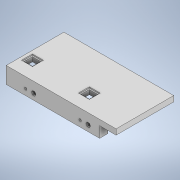
# Autodesk Inventor part: side_bumper_lower_R_new
Saved by Autodesk Inventor 2020 (Build 240168000, 168)
## iProperties
Created: 2022-10-31
Part Number: side_bumper_lower_R_new
Material: 일반
Document SubType Name: Modeling
Designer: SeungJin
Density: 1 g/cm^3
Appearance: 기본값
Author: SeungJin
Autodesk Inventor part; units mm, degrees
ref_plane "YZ Plane" through (0, 0, 0) normal (1, 0, 0) x (0, 1, 0)
ref_plane "XZ Plane" through (0, 0, 0) normal (0, 1, 0) x (-1, 0, 0)
ref_plane "작업 평면1" through (18.73, 22.5444, -43) normal (0, 0, -1) x (-1, 0, 0)
sketch "스케치1" plane through (18.73, 22.5444, -43) normal (0, 0, -1) x (-1, 0, 0)
  circle A0 centre (15, -32.544) radius 4
  circle A1 centre (215, -32.544) radius 4
  circle A2 centre (164.635, -19) radius 2.25
  circle A3 centre (65.365, -19) radius 2.25
  line L0 (230, 0) -> (230, -40)
  line L1 (0, 0) -> (230, 0)
  line L2 (0, -40) -> (0, 0)
  line L3 (230, -40) -> (0, -40)
  line L4 (230, -40) -> (0, -40)
  line L5 (0, 0) -> (230, 0)
  line L6 (200, -40) -> (200, 0)
  line L7 (30, -40) -> (30, 0)
  line L8 (230, -10) -> (0, -10)
  point P0 (200, 0)
  point P1 (30, -10)
  dimension "d5" = 40
  dimension "d6" = 230
  dimension "d7" = 15
  dimension "d8" = 7.456
  dimension "d9" = 7.456
  dimension "d10" = 15
  dimension "d11" = 19
  dimension "d12" = 19
  dimension "d13" = 65.365
  dimension "d14" = 65.365
  dimension "d22" = 30
  dimension "d23" = 30
  dimension "d24" = 10
  constraints: 18 end point, 7 centre point, 6 perpendicular, 6 point on line
  measures "d5" distance of L2.start L1.start
  measures "d6" distance of L0.end L2.start
  measures "d7" distance from line of L2 A0.centre
  measures "d8" distance from line of L3 A0.centre
  measures "d9" distance from line of L3 A1.centre
  measures "d10" distance from line of L0 A1.centre
  measures "d11" distance from line of L1 A3.centre
  measures "d12" distance from line of L1 A2.centre
  measures "d13" distance from line of L0 A2.centre
  measures "d14" distance from line of L2 A3.centre
  measures "d22" distance between parallel lines of L6 L0
  measures "d23" distance between parallel lines of L2 L7
  measures "d24" distance between parallel lines of L1 L8
extrude "돌출1" add sketch "스케치1" along normal blind 15 contours L6 L8 L7 L1 | L6 L3 L7 L8 | L7 L8 L2 L1
sketch "스케치2" plane through (18.73, 22.5444, -58) normal (0, 0, -1) x (-1, 0, 0)
  line L0 (30, -40) -> (200, -40) projected
  line L1 (200, 0) -> (0, 0) projected
  line L2 (0, 0) -> (0, -10) projected
  circle A0 centre (164.635, -19) radius 2.25 projected
  circle A1 centre (65.365, -19) radius 2.25 projected
  line L3 (0, -10) -> (200, -10)
  line L4 (200, -40) -> (200, 0) projected
  line L5 (0, -10) -> (30, -10) projected
  line L6 (30, -10) -> (30, -40) projected
  point P0 (18.73, -22.5444)
  dimension "d15" = 10
  constraints: 2 end point, 2 point on line
  measures "d15" distance between parallel lines of L1 L3
extrude "돌출2" add sketch "스케치2" along normal blind 90 contours L3 L2 L1 L4
sketch "스케치3" plane through (18.73, 22.5444, -58) normal (0, 0, -1) x (-1, 0, 0)
  circle A0 centre (65.365, -19) radius 2.25 projected
  circle A1 centre (164.635, -19) radius 2.25 projected
  circle A2 centre (65.365, -19) radius 3.6
  circle A3 centre (164.635, -19) radius 3.6
  line L0 (162.5565, -22.6) -> (160.4781, -19)
  line L1 (160.4781, -19) -> (162.5565, -15.4)
  line L2 (162.5565, -15.4) -> (166.7134, -15.4)
  line L3 (166.7134, -15.4) -> (168.7919, -19)
  line L4 (168.7919, -19) -> (166.7134, -22.6)
  line L5 (166.7134, -22.6) -> (162.5565, -22.6)
  line L6 (63.2866, -22.6) -> (61.2081, -19)
  line L7 (61.2081, -19) -> (63.2866, -15.4)
  line L8 (63.2866, -15.4) -> (67.4435, -15.4)
  line L9 (67.4435, -15.4) -> (69.5219, -19)
  line L10 (69.5219, -19) -> (67.4435, -22.6)
  line L11 (67.4435, -22.6) -> (63.2866, -22.6)
  point P0 (18.73, -22.5444)
  point P1 (164.635, -22.6)
  point P2 (65.365, -22.6)
  dimension "d18" = 7.2
  dimension "d19" = 7.2
  constraints: 24 end point, 4 coincident, 2 midpoint, 2 vertical alignment, 1 point on line, 30 other
extrude "돌출3" cut sketch "스케치3" against normal blind 12 contours A0 | A1 | A2 | A2 L9 L10 | A2 L8 L9 | L10 L11 A2 | A2 L7 L8 | L11 L6 A2 | A2 L6 L7 | A3 | A3 L3 L4 | A3 L2 L3 | L4 L5 A3 | A3 L1 L2 | L5 L0 A3 | A3 L0 L1
sketch "스케치4" plane through (18.73, 22.5444, -58) normal (0, 0, -1) x (-1, 0, 0)
  line L0 (162.5565, -22.6) -> (160.4781, -19) projected
  line L1 (160.4781, -19) -> (162.5565, -15.4) projected
  line L2 (162.5565, -15.4) -> (166.7134, -15.4) projected
  line L3 (166.7134, -15.4) -> (168.7919, -19) projected
  line L4 (168.7919, -19) -> (166.7134, -22.6) projected
  line L5 (166.7134, -22.6) -> (162.5565, -22.6) projected
  line L6 (61.2081, -19) -> (63.2866, -15.4) projected
  line L7 (63.2866, -15.4) -> (67.4435, -15.4) projected
  line L8 (67.4435, -15.4) -> (69.5219, -19) projected
  line L9 (69.5219, -19) -> (67.4435, -22.6) projected
  line L10 (67.4435, -22.6) -> (63.2866, -22.6) projected
  line L11 (63.2866, -22.6) -> (61.2081, -19) projected
  line L12 (200, -10) -> (30, -10) projected
  line L13 (30, -10) -> (30, -40) projected
  line L14 (30, -40) -> (200, -40) projected
  line L15 (200, -40) -> (200, -10) projected
  circle A0 centre (164.635, -19) radius 2.25 projected
  circle A1 centre (65.365, -19) radius 2.25 projected
  point P0 (18.73, -22.5444)
  point P1 (50.73, -19)
  point P2 (150, -19)
  dimension "d25" = 14.635
  dimension "d26" = 14.635
  constraints: 2 horizontal alignment
  measures "d25" distance of point (65.365, -19) point (50.73, -19)
  measures "d26" distance of A0.centre point (150, -19)
hole "구멍1" at (-32, 3.5444, -58) at (-131.2699, 3.5444, -58) direction (0, 0, 1) diameter 4.5 end through all clearance for "Hex Head Cap Screw ISO 24017" size "M4" standard "ISO"
sketch "스케치5" plane through (18.73, 22.5444, -43) normal (0, 0, 1) x (1, 0, 0)
  circle A0 centre (-50.73, -19) radius 2.25 projected
  circle A1 centre (-150, -19) radius 2.25 projected
  line L0 (-30, -40) -> (-200, -40) projected
  line L1 (-30, -10) -> (-30, -40) projected
  line L2 (0, -10) -> (-30, -10) projected
  line L3 (0, 0) -> (0, -10) projected
  line L4 (-200, 0) -> (0, 0) projected
  line L5 (-200, -40) -> (-200, 0) projected
  circle A2 centre (-164.635, -19) radius 2.25 projected
  circle A3 centre (-65.365, -19) radius 2.25 projected
  circle A4 centre (-150, -19) radius 2.25 projected
  circle A5 centre (-150, -19) radius 3.6
  circle A6 centre (-50.73, -19) radius 2.25 projected
  circle A7 centre (-50.73, -19) radius 3.6
  line L6 (-147.9215, -15.4) -> (-145.8431, -19)
  line L7 (-145.8431, -19) -> (-147.9215, -22.6)
  line L8 (-147.9215, -22.6) -> (-152.0784, -22.6)
  line L9 (-152.0784, -22.6) -> (-154.1569, -19)
  line L10 (-154.1569, -19) -> (-152.0784, -15.4)
  line L11 (-152.0784, -15.4) -> (-147.9215, -15.4)
  line L12 (-48.6516, -15.4) -> (-46.5731, -19)
  line L13 (-46.5731, -19) -> (-48.6516, -22.6)
  line L14 (-48.6516, -22.6) -> (-52.8085, -22.6)
  line L15 (-52.8085, -22.6) -> (-54.8869, -19)
  line L16 (-54.8869, -19) -> (-52.8085, -15.4)
  line L17 (-52.8085, -15.4) -> (-48.6516, -15.4)
  point P0 (-18.73, -22.5444)
  point P1 (-150, -15.4)
  point P2 (-50.73, -15.4)
  dimension "d34" = 7.2
  dimension "d35" = 7.2
  constraints: 24 end point, 4 coincident, 2 midpoint, 2 vertical alignment, 1 point on line, 30 other
extrude "돌출4" cut sketch "스케치5" against normal blind 12 contours A0 | A1 | A5 | A5 L6 L7 | A5 L11 L6 | L7 L8 A5 | A5 L10 L11 | L8 L9 A5 | A5 L9 L10 | A7 | A7 L12 L13 | A7 L17 L12 | L13 L14 A7 | A7 L16 L17 | L14 L15 A7 | A7 L15 L16
sketch "스케치6" plane through (-181.27, 22.5444, -43) normal (0, 1, 0) x (1, 0, 0)
  line L0 (147.02, 12) -> (151.52, 12) projected
  line L1 (0, 0) -> (200, 0) projected
  line L2 (200, 0) -> (200, 105) projected
  line L3 (0, 105) -> (200, 105) projected
  line L4 (0, 0) -> (0, 105) projected
  line L5 (0, 0) -> (200, 0) projected
  line L6 (129.27, 0) -> (129.27, 105)
  line L7 (200, 105) -> (0, 105) projected
  line L8 (47.75, 12) -> (52.25, 12) projected
  line L9 (47.9216, 12) -> (52.0785, 12) projected
  line L10 (25.73, 0) -> (25.73, 105)
  line L11 (200, 22) -> (0, 22)
  line L12 (0, 15) -> (0, 105) projected
  line L13 (129.27, 22) -> (109.27, 22)
  line L14 (109.27, 22) -> (109.27, 42)
  line L15 (109.27, 42) -> (129.27, 42)
  line L16 (129.27, 42) -> (129.27, 22)
  line L17 (25.73, 22) -> (5.73, 22)
  line L18 (5.73, 22) -> (5.73, 42)
  line L19 (5.73, 42) -> (25.73, 42)
  line L20 (25.73, 42) -> (25.73, 22)
  point P0 (181.27, -43)
  point P1 (149.27, 12)
  point P2 (50, 12)
  point P3 (25.73, 42)
  point P4 (109.27, 22)
  dimension "d38" = 20
  dimension "d39" = 24.27
  dimension "d40" = 22
  dimension "d41" = 20
  dimension "d42" = 20
  dimension "d43" = 20
  dimension "d44" = 20
  constraints: 22 end point, 10 point on line, 4 parallel, 3 horizontal, 3 perpendicular, 2 midpoint, 1 vertical
  measures "d38" distance from line of point (149.27, 12) L6
  measures "d39" distance from line of L10 point (50, 12)
  measures "d40" distance between parallel lines of L11 L1
  measures "d41" distance of L14.end L15.end
  measures "d42" distance of L13.end L14.end
  measures "d43" distance of L18.end L19.end
  measures "d44" distance of L17.end L18.end
extrude "돌출5" cut sketch "스케치6" against normal blind 2 contours L11 L18 L19 L10 | L11 L14 L15 L6
sketch "스케치7" plane through (-181.27, 20.5444, -43) normal (0, 1, 0) x (1, 0, 0)
  line L0 (109.27, 42) -> (129.27, 42) projected
  line L1 (109.27, 22) -> (109.27, 42) projected
  line L2 (129.27, 22) -> (109.27, 22) projected
  line L3 (129.27, 42) -> (129.27, 22) projected
  line L4 (5.73, 22) -> (5.73, 42) projected
  line L5 (25.73, 22) -> (5.73, 22) projected
  line L6 (25.73, 42) -> (25.73, 22) projected
  line L7 (5.73, 42) -> (25.73, 42) projected
  line L8 (126.77, 24.5) -> (111.77, 24.5)
  line L9 (111.77, 24.5) -> (111.77, 39.5)
  line L10 (111.77, 39.5) -> (126.77, 39.5)
  line L11 (126.77, 39.5) -> (126.77, 24.5)
  line L12 (126.77, 24.5) -> (111.77, 39.5) construction
  line L13 (111.77, 24.5) -> (126.77, 39.5) construction
  line L14 (23.23, 24.5) -> (8.23, 24.5)
  line L15 (8.23, 24.5) -> (8.23, 39.5)
  line L16 (8.23, 39.5) -> (23.23, 39.5)
  line L17 (23.23, 39.5) -> (23.23, 24.5)
  line L18 (23.23, 24.5) -> (8.23, 39.5) construction
  line L19 (8.23, 24.5) -> (23.23, 39.5) construction
  point P0 (181.27, -43)
  point P1 (119.27, 32)
  point P2 (15.73, 32)
  dimension "d47" = 15
  dimension "d48" = 15
  dimension "d49" = 15
  dimension "d50" = 15
  constraints: 24 end point, 4 midpoint, 4 parallel, 2 horizontal, 2 perpendicular
  measures "d47" distance of L9.end L10.end
  measures "d48" distance of L8.end L9.end
  measures "d49" distance of L15.end L16.end
  measures "d50" distance of L14.end L15.end
extrude "돌출6" cut sketch "스케치7" against normal through all contours L8 L9 L10 L11 | L14 L15 L16 L17
sketch "스케치8" plane through (-181.27, -17.4556, -43) normal (0, -1, 0) x (1, 0, 0)
  line L0 (170, 0) -> (0, 0) projected
  line L1 (0, 0) -> (0, -15) projected
  line L2 (170, -15) -> (0, -15) projected
  line L3 (170, 0) -> (170, -15) projected
  line L4 (52.25, -12) -> (47.75, -12) projected
  line L5 (151.52, -12) -> (147.02, -12) projected
  line L6 (170, 0) -> (0, 0) projected
  line L7 (149.27, -15) -> (149.27, 0)
  line L8 (21.27, 0) -> (21.27, -15)
  line L9 (21.27, -7.5) -> (149.27, -7.5)
  line L10 (0, -15) -> (170, -15) projected
  line L11 (5.27, 0) -> (165.27, 0)
  line L12 (165.27, 0) -> (165.27, -15)
  line L13 (165.27, -15) -> (5.27, -15)
  line L14 (5.27, -15) -> (5.27, 0)
  point P0 (181.27, 43)
  point P1 (149.27, 0)
  point P2 (39.5219, -15)
  point P3 (21.27, 0)
  point P4 (85.27, -7.5)
  dimension "d56" = 128
  dimension "d57" = 160
  constraints: 14 end point, 5 point on line, 3 midpoint, 2 parallel, 2 perpendicular, 1 horizontal, 1 vertical, 1 other
  measures "d56" distance between parallel lines of L8 L7
  measures "d57" distance of L12.end L13.end
extrude "돌출7" cut sketch "스케치8" against normal blind 10
equation "\"d3\" = d7"
